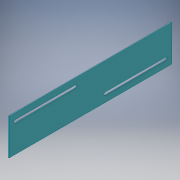
# Autodesk Inventor part: 6 x 27 x 1+8
Saved by Autodesk Inventor 2016 (Build 200138000, 138)
## iProperties
Created: 2015-06-18
Part Number: 6 x 27 x 1+8
Material: Aluminum 6061
Document SubType Name: Modeling
Designer: steele
Density: 2.7 g/cm^3
Appearance: Cadet Blue
Mass: 838.485 g
Surface Area: 2044.24 cm^2
Volume: 310.55 cm^3
Author: steele
Autodesk Inventor part; units mm, degrees
ref_plane "YZ Plane" through (0, 0, 0) normal (1, 0, 0) x (0, 1, 0)
ref_plane "XZ Plane" through (0, 0, 0) normal (0, 1, 0) x (-1, 0, 0)
ref_plane "XY Plane" through (0, 0, 0) normal (0, 0, 1) x (1, 0, 0)
sketch "Sketch1" plane through (0, 0, 0) normal (1, 0, 0) x (0, 1, 0)
  line L0 (-76.2, 342.9) -> (-76.2, -342.9)
  line L1 (-76.2, -342.9) -> (76.2, -342.9)
  line L2 (76.2, -342.9) -> (76.2, 342.9)
  line L3 (76.2, 342.9) -> (-76.2, 342.9)
  line L4 (-76.2, 342.9) -> (76.2, -342.9) construction
  line L5 (-76.2, -342.9) -> (76.2, 342.9) construction
  point P0 (0, 0)
  dimension "width" = 685.8
  dimension "height" = 152.4
  constraints: 12 end point, 2 midpoint, 2 parallel, 1 perpendicular, 1 vertical
  measures "width" distance of L0.start L0.end
  measures "height" distance of L0.end L1.end
extrude "Extrusion1" add sketch "Sketch1" along normal blind 3.175
sketch "Sketch2" plane through (3.175, 0, 0) normal (1, 0, 0) x (0, 0, -1)
  line L0 (-317.5, 44.45) -> (-63.5, 44.45) construction
  line L1 (-317.5, 38.1) -> (-63.5, 38.1)
  line L2 (-63.5, 50.8) -> (-317.5, 50.8)
  arc A0 (-317.5, 50.8) -> (-317.5, 38.1) centre (-317.5, 44.45) ccw
  arc A1 (-63.5, 38.1) -> (-63.5, 50.8) centre (-63.5, 44.45) ccw
  line L3 (342.9, 76.2) -> (-342.9, 76.2) projected
  line L4 (-342.9, 76.2) -> (-342.9, -76.2) projected
  line L5 (63.5, -44.45) -> (317.5, -44.45) construction
  line L6 (63.5, -50.8) -> (317.5, -50.8)
  line L7 (317.5, -38.1) -> (63.5, -38.1)
  arc A2 (63.5, -38.1) -> (63.5, -50.8) centre (63.5, -44.45) ccw
  arc A3 (317.5, -50.8) -> (317.5, -38.1) centre (317.5, -44.45) ccw
  line L8 (-342.9, -76.2) -> (342.9, -76.2) projected
  line L9 (342.9, -76.2) -> (342.9, 76.2) projected
  point P0 (0, 0)
  point P1 (-190.5, 44.45)
  point P2 (190.5, -44.45)
  dimension "slot_center_from_top" = 31.75
  dimension "slot_center_from_side" = 152.4
  dimension "slot_radius" = 6.35
  dimension "d7" = 31.75
  dimension "d8" = 152.4
  dimension "d9" = 6.35
  dimension "length_of_slot" = 254
  dimension "d13" = 254
  constraints: 16 end point, 8 point on circle, 8 tangent, 4 centre point, 2 horizontal, 2 midpoint, 2 parallel
  measures "slot_center_from_top" distance from line of point (-190.5, 44.45) L3
  measures "slot_center_from_side" distance from line of point (-190.5, 44.45) L4
  measures "slot_radius" radius of A1
  measures "d7" distance from line of point (190.5, -44.45) L8
  measures "d8" distance from line of point (190.5, -44.45) L9
  measures "d9" radius of A2
  measures "length_of_slot" distance of L0.start L0.end
  measures "d13" distance of L5.start L5.end
extrude "Extrusion2" cut sketch "Sketch2" against normal through all contours A0 L2 A1 L1 | A2 L7 A3 L6
equation "\"d7\" = slot_center_from_top"
equation "\"d8\" = slot_center_from_side"
equation "\"d9\" = slot_radius"
equation "\"d13\" = length_of_slot"
body "Solid1"
